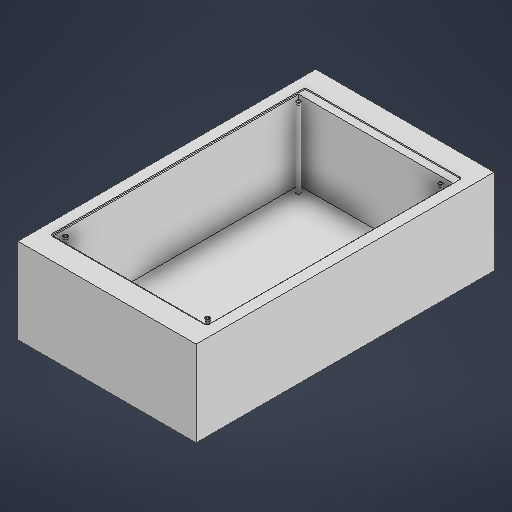
# Autodesk Inventor part: Enclosure
Saved by Autodesk Inventor 2025.2 (Build 292293000, 293)
## iProperties
Created: 2025-02-10
Part Number: Enclosure
Material: Generic
Document SubType Name: Modeling
Designer: elier
Density: 1 g/cm^3
Appearance: Default
Author: elier
Autodesk Inventor part; units mm, degrees
ref_plane "YZ Plane" through (0, 0, 0) normal (1, 0, 0) x (0, 1, 0)
ref_plane "XZ Plane" through (0, 0, 0) normal (0, 1, 0) x (-1, 0, 0)
ref_plane "XY Plane" through (0, 0, 0) normal (0, 0, 1) x (1, 0, 0)
sketch "Sketch1" plane through (0, 0, 0) normal (0, 1, 0) x (-1, 0, 0)
  line L0 (-83.5, 139.5) -> (83.5, 139.5)
  line L1 (83.5, 139.5) -> (83.5, -139.5)
  line L2 (83.5, -139.5) -> (-83.5, -139.5)
  line L3 (-83.5, -139.5) -> (-83.5, 139.5)
  line L4 (-83.5, 139.5) -> (83.5, -139.5) construction
  line L5 (83.5, 139.5) -> (-83.5, -139.5) construction
  point P0 (0, 0)
  dimension "d0" = 167
  dimension "d1" = 279
  constraints: 12 end point, 2 midpoint, 2 parallel, 1 horizontal, 1 perpendicular
  measures "d0" distance of L1.end L2.end
  measures "d1" distance of L0.end L1.end
extrude "Extrusion1" add sketch "Sketch1" along normal blind 80
sketch "Sketch2" plane through (0, 80, 0) normal (0, 1, 0) x (1, 0, 0)
  line L0 (71.5, -119.5) -> (-71.5, -119.5)
  line L1 (-73.5, -117.5) -> (-73.5, 117.5)
  line L2 (-71.5, 119.5) -> (71.5, 119.5)
  line L3 (73.5, 117.5) -> (73.5, -117.5)
  line L4 (73.5, -119.5) -> (-73.5, 119.5) construction
  line L5 (-73.5, -119.5) -> (73.5, 119.5) construction
  arc A0 (-73.5, -117.5) -> (-71.5, -119.5) centre (-71.5, -117.5) ccw
  arc A1 (-71.5, 119.5) -> (-73.5, 117.5) centre (-71.5, 117.5) ccw
  arc A2 (73.5, 117.5) -> (71.5, 119.5) centre (71.5, 117.5) ccw
  arc A3 (71.5, -119.5) -> (73.5, -117.5) centre (71.5, -117.5) ccw
  point P0 (0, 0)
  dimension "d4" = 147
  dimension "d5" = 239
  dimension "d6" = 2
  constraints: 12 end point, 8 point on circle, 8 point on line, 8 tangent, 4 centre point, 3 equal radius, 2 midpoint, 2 parallel, 1 horizontal, 1 perpendicular
  measures "d4" distance of L4.end L5.end
  measures "d5" distance of L5.start L4.end
  measures "d6" radius of A0
extrude "Extrusion2" cut sketch "Sketch2" against normal blind 1.1
sketch "Sketch3" plane through (0, 78.9, 0) normal (0, 1, 0) x (1, 0, 0)
  line L0 (-73.5, -117.5) -> (-73.5, 117.5) projected
  line L1 (71.5, -119.5) -> (-71.5, -119.5) projected
  line L2 (-72.25, -117.83) -> (72.25, -117.83)
  line L3 (72.25, -117.83) -> (72.25, 112.27)
  line L4 (72.25, 112.27) -> (-72.25, 112.27)
  line L5 (-72.25, 112.27) -> (-72.25, -117.83)
  point P0 (0, 0)
  dimension "d9" = 1.25
  dimension "d10" = 1.67
  dimension "d11" = 144.5
  dimension "d12" = 230.1
  constraints: 8 end point, 2 parallel, 1 horizontal, 1 perpendicular
  measures "d9" distance from line of L0 L2.start
  measures "d10" distance from line of L1 L2.start
  measures "d11" distance of L4.end L3.end
  measures "d12" distance of L3.end L2.end
extrude "Extrusion3" cut sketch "Sketch3" against normal blind 73.9
sketch "Sketch4" plane through (0, 5, 0) normal (0, 1, 0) x (1, 0, 0)
  circle A0 centre (-66.5, -111.83) radius 2
  line L0 (72.25, -117.83) -> (-72.25, -117.83) projected
  line L1 (-72.25, -117.83) -> (-72.25, 112.27) projected
  circle A1 centre (66.5, -111.83) radius 2
  line L2 (72.25, 112.27) -> (72.25, -117.83) projected
  circle A2 centre (-66.5, 106.27) radius 2
  line L3 (-72.25, 112.27) -> (72.25, 112.27) projected
  circle A3 centre (66.5, 106.27) radius 2
  point P0 (0, 0)
  dimension "d15" = 4
  dimension "d16" = 6
  dimension "d17" = 5.75
  dimension "d18" = 4
  dimension "d19" = 6
  dimension "d20" = 5.75
  dimension "d21" = 4
  dimension "d22" = 5.75
  dimension "d23" = 6
  dimension "d24" = 4
  dimension "d25" = 6
  dimension "d26" = 5.75
  constraints: 4 centre point
  measures "d15" diameter of A0
  measures "d16" distance from line of L0 A0.centre
  measures "d17" distance from line of L1 A0.centre
  measures "d18" diameter of A1
  measures "d19" distance from line of L0 A1.centre
  measures "d20" distance from line of L2 A1.centre
  measures "d21" diameter of A2
  measures "d22" distance from line of L1 A2.centre
  measures "d23" distance from line of L3 A2.centre
  measures "d24" diameter of A3
  measures "d25" distance from line of L3 A3.centre
  measures "d26" distance from line of L2 A3.centre
extrude "Extrusion4" add sketch "Sketch4" along normal blind 73.9 contours A0 | A1 | A2 | A3
sketch "Sketch5" plane through (0, 5, 0) normal (0, 1, 0) x (1, 0, 0)
  circle A0 centre (-66.5, -111.83) radius 2 projected
  circle A1 centre (-66.5, -111.83) radius 1.25
  circle A2 centre (-66.5, 106.27) radius 2 projected
  circle A3 centre (-66.5, 106.27) radius 1.25
  circle A4 centre (66.5, 106.27) radius 2 projected
  circle A5 centre (66.5, 106.27) radius 1.25
  circle A6 centre (66.5, -111.83) radius 1.25
  point P0 (0, 0)
  dimension "d29" = 2.5
  dimension "d30" = 2.5
  dimension "d31" = 2.5
  dimension "d32" = 2.5
  constraints: 4 centre point, 3 coincident
  measures "d29" diameter of A1
  measures "d30" diameter of A3
  measures "d31" diameter of A5
  measures "d32" diameter of A6
extrude "Extrusion5" cut sketch "Sketch5" along normal blind 73.9 and the other way blind 5 contours A1 | A3 | A5 | A6
sketch "Sketch6" plane through (0, 0, 0) normal (0, -1, 0) x (1, 0, 0)
  circle A0 centre (-66.5, -106.27) radius 1.25 projected
  circle A1 centre (-66.5, -106.27) radius 1.75
  circle A2 centre (-66.5, 111.83) radius 1.25 projected
  circle A3 centre (-66.5, 111.83) radius 1.75
  circle A4 centre (66.5, 111.83) radius 1.25 projected
  circle A5 centre (66.5, 111.83) radius 1.75
  circle A6 centre (66.5, -106.27) radius 1.25 projected
  circle A7 centre (66.5, -106.27) radius 1.75
  point P0 (0, 0)
  dimension "d37" = 3.5
  dimension "d38" = 3.5
  dimension "d39" = 3.5
  dimension "d40" = 3.5
  constraints: 4 centre point, 4 coincident
  measures "d37" diameter of A1
  measures "d38" diameter of A3
  measures "d39" diameter of A5
  measures "d40" diameter of A7
extrude "Extrusion6" cut sketch "Sketch6" against normal blind 76.9 contours A0 | A1 | A2 | A3 | A4 | A5 | A6 | A7
body "Solid1"
